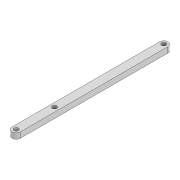
# Autodesk Inventor part: Part_2
Saved by Autodesk Inventor 2022 (Build 260153000, 153)
## iProperties
Created: 2022-04-22
Part Number: Part_2
Material: Generic
Document SubType Name: Modeling
Designer: dell
Density: 1 g/cm^3
Appearance: Default
Author: dell
Autodesk Inventor part; units mm, degrees
ref_plane "YZ Plane" through (0, 0, 0) normal (1, 0, 0) x (0, 1, 0)
ref_plane "XZ Plane" through (0, 0, 0) normal (0, 1, 0) x (-1, 0, 0)
ref_plane "XY Plane" through (0, 0, 0) normal (0, 0, 1) x (1, 0, 0)
sketch "Sketch1" plane through (0, 0, 0) normal (0, 1, 0) x (-1, 0, 0)
  line L0 (0, 0) -> (0, -105.413) construction
  line L1 (3, 0) -> (3, -105.413)
  line L2 (-3, -105.413) -> (-3, 0)
  arc A0 (3, 0) -> (-3, 0) centre (0, 0) ccw
  arc A1 (-3, -105.413) -> (3, -105.413) centre (0, -105.413) ccw
  circle A2 centre (0, 0) radius 1.6
  circle A3 centre (0, -105.413) radius 1.6
  circle A4 centre (0, -27.392) radius 1.6
  point P0 (0, -52.7065)
  dimension "d0" = 3.2
  dimension "d1" = 3.2
  dimension "d2" = 6
  dimension "d3" = 105.413
  dimension "d4" = 3.2
  dimension "d5" = 27.392
  constraints: 8 end point, 5 centre point, 4 point on circle, 4 tangent, 2 coincident, 1 midpoint, 1 parallel, 1 point on line, 1 vertical
  measures "d0" diameter of A2
  measures "d1" diameter of A3
  measures "d2" distance between parallel lines of L2 L1
  measures "d3" distance of L0.end L0.start
  measures "d4" diameter of A4
  measures "d5" distance of L0.start A4.centre
extrude "Extrusion1" add sketch "Sketch1" along normal blind 4
body "Solid1"
